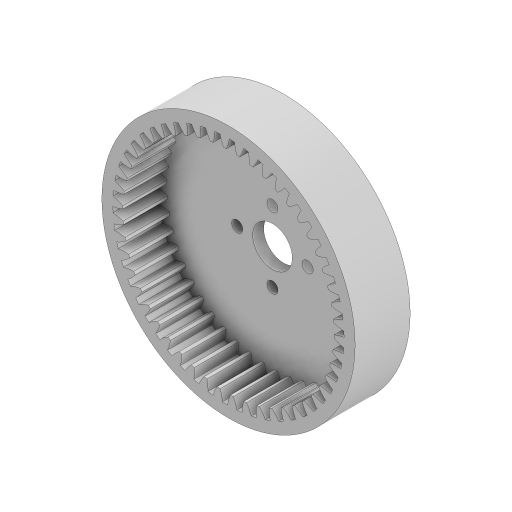
# Autodesk Inventor part: PLANETARIO CORONA
Saved by Autodesk Inventor 2024 (Build 280153000, 153)
## iProperties
Created: 2024-06-18
Part Number: PLANETARIO CORONA
Material: Generic
Document SubType Name: Modeling
Designer: Jhuliams
Density: 1 g/cm^3
Appearance: Default
Author: Jhuliams
Autodesk Inventor part; units mm, degrees
ref_plane "YZ Plane" through (0, 0, 0) normal (1, 0, 0) x (0, 1, 0)
ref_plane "XZ Plane" through (0, 0, 0) normal (0, 1, 0) x (-1, 0, 0)
ref_plane "XY Plane" through (0, 0, 0) normal (0, 0, 1) x (1, 0, 0)
sketch "Sketch1" plane through (0, 0, 0) normal (0, 0, 1) x (1, 0, 0)
  circle A0 centre (0, 0) radius 52.5
  arc A1 (47.9537, -2.1069) -> (47.994, -0.7575) centre (0, 0) ccw
  line L0 (0, 0) -> (74.2646, 0) construction
  line L1 (0, 0) -> (65.7808, 0) construction
  arc A2 (36.3859, -31.306) -> (40.9396, -32.8664) centre (44.1511, -16.0697) ccw
  arc A3 (47.9537, -2.1069) -> (52.3718, -3.6673) centre (55.8044, 13.0856) ccw
  arc A4 (52.4973, 0.5366) -> (47.994, -0.7575) centre (54.9244, -16.3913) ccw
  arc A5 (47.8397, 3.9199) -> (47.7105, 5.2637) centre (0, 0) ccw
  arc A6 (47.8397, 3.9199) -> (52.4184, 2.9255) centre (53.7243, 19.9766) ccw
  arc A7 (52.016, 7.112) -> (47.7105, 5.2637) centre (56.5456, -9.3782) ccw
  arc A8 (46.9711, 9.8849) -> (46.6746, 11.2019) centre (0, 0) ccw
  arc A9 (46.9711, 9.8849) -> (51.6384, 9.4722) centre (50.7969, 26.5525) ccw
  arc A10 (50.7145, 13.5753) -> (46.6746, 11.2019) centre (57.2752, -2.2172) ccw
  arc A11 (45.3619, 15.694) -> (44.9026, 16.9634) centre (0, 0) ccw
  arc A12 (45.3619, 15.694) -> (50.0441, 15.8695) centre (47.0684, 32.7097) ccw
  arc A13 (48.6132, 19.8244) -> (44.9026, 16.9634) centre (57.1014, 4.9787) ccw
  arc A14 (43.0372, 21.2556) -> (42.4224, 22.4575) centre (0, 0) ccw
  arc A15 (43.0372, 21.2556) -> (47.6605, 22.0166) centre (42.5977, 38.351) ccw
  arc A16 (45.7452, 25.761) -> (42.4224, 22.4575) centre (56.0272, 12.0962) ccw
  arc A17 (40.0338, 26.482) -> (39.2732, 27.5973) centre (0, 0) ccw
  arc A18 (40.0338, 26.482) -> (44.5252, 27.8164) centre (37.4551, 43.3875) ccw
  arc A19 (42.1558, 31.2912) -> (39.2732, 27.5973) centre (54.0693, 19.0229) ccw
  arc A20 (36.399, 31.2907) -> (35.5047, 32.3019) centre (0, 0) ccw
  arc A21 (36.399, 31.2907) -> (40.6878, 33.1776) centre (31.7219, 47.7397) ccw
  arc A22 (37.9015, 36.328) -> (35.5047, 32.3019) centre (51.2588, 25.6496) ccw
  arc A23 (32.1902, 35.606) -> (31.1762, 36.4972) centre (0, 0) ccw
  arc A24 (32.1902, 35.606) -> (36.2087, 38.0155) centre (25.4884, 51.3391) ccw
  arc A25 (33.0496, 40.7919) -> (31.1762, 36.4972) centre (47.6398, 31.8717) ccw
  arc A26 (27.4738, 39.3598) -> (26.3561, 40.1168) centre (0, 0) ccw
  arc A27 (27.4738, 39.3598) -> (31.1586, 42.2539) centre (18.8529, 54.1288) ccw
  arc A28 (27.6764, 44.6124) -> (26.3561, 40.1168) centre (43.2696, 37.5913) ccw
  arc A29 (22.3241, 42.4928) -> (21.1203, 43.1037) centre (0, 0) ccw
  arc A30 (22.3241, 42.4928) -> (25.6171, 45.8259) centre (11.9201, 56.0649) ccw
  arc A31 (21.8667, 47.7294) -> (21.1203, 43.1037) centre (38.217, 42.718) ccw
  arc A32 (16.8223, 44.9557) -> (15.5514, 45.4109) centre (0, 0) ccw
  arc A33 (16.8223, 44.9557) -> (19.6716, 48.6752) centre (4.7993, 57.1168) ccw
  arc A34 (15.7122, 50.0937) -> (15.5514, 45.4109) centre (32.5616, 47.171) ccw
  arc A35 (11.0552, 46.7096) -> (9.7373, 47.002) centre (0, 0) ccw
  arc A36 (11.0552, 46.7096) -> (13.4159, 50.7569) centre (-2.3971, 57.2679) ccw
  arc A37 (9.3099, 51.6679) -> (9.7373, 47.002) centre (26.3928, 50.8801) ccw
  arc A38 (5.1138, 47.7268) -> (3.7696, 47.8518) centre (0, 0) ccw
  arc A39 (5.1138, 47.7268) -> (6.9486, 52.0381) centre (-9.5558, 56.5159) ccw
  arc A40 (2.7608, 52.4274) -> (3.7696, 47.8518) centre (19.8077, 53.7868) ccw
  arc A41 (-0.9083, 47.9914) -> (-2.2575, 47.9469) centre (0, 0) ccw
  arc A42 (-0.9083, 47.9914) -> (0.3717, 52.4987) centre (-16.5638, 54.8726) ccw
  arc A43 (-3.8319, 52.36) -> (-2.2575, 47.9469) centre (12.9102, 55.8452) ccw
  arc A44 (-6.9161, 47.4991) -> (-8.2491, 47.2859) centre (0, 0) ccw
  arc A45 (-6.9161, 47.4991) -> (-6.2111, 52.1313) centre (-23.3105, 52.3639) ccw
  arc A46 (-10.3641, 51.4668) -> (-8.2491, 47.2859) centre (5.8092, 57.0229) ccw
  arc A47 (-12.8148, 46.2578) -> (-14.1105, 45.8791) centre (0, 0) ccw
  arc A48 (-12.8148, 46.2578) -> (-12.6959, 50.9418) centre (-29.6897, 49.0294) ccw
  arc A49 (-16.7329, 49.762) -> (-14.1105, 45.8791) centre (-1.3835, 57.3014) ccw
  arc A50 (-18.5113, 44.2869) -> (-19.7494, 43.7488) centre (0, 0) ccw
  arc A51 (-18.5113, 44.2869) -> (-18.9805, 48.9489) centre (-35.6006, 44.9217) ccw
  arc A52 (-22.8378, 47.2725) -> (-19.7494, 43.7488) centre (-8.5543, 56.6761) ccw
  arc A53 (-23.916, 41.6176) -> (-25.0769, 40.9286) centre (0, 0) ccw
  arc A54 (-23.916, 41.6176) -> (-24.9658, 46.184) centre (-40.95, 40.1055) ccw
  arc A55 (-28.5825, 44.0374) -> (-25.0769, 40.9286) centre (-15.5903, 55.1571) ccw
  arc A56 (-28.9435, 38.292) -> (-30.0088, 37.4629) centre (0, 0) ccw
  arc A57 (-28.9435, 38.292) -> (-30.5573, 42.6908) centre (-45.6537, 34.6569) ccw
  arc A58 (-33.8765, 40.1078) -> (-30.0088, 37.4629) centre (-22.3804, 52.7682) ccw
  arc A59 (-33.5145, 34.3624) -> (-34.4676, 33.4064) centre (0, 0) ccw
  arc A60 (-33.5145, 34.3624) -> (-35.6669, 38.5243) centre (-49.6373, 28.6617) ccw
  arc A61 (-38.6362, 35.5457) -> (-34.4676, 33.4064) centre (-28.8175, 49.5471) ccw
  arc A62 (-37.557, 29.891) -> (-38.3827, 28.823) centre (0, 0) ccw
  arc A63 (-37.557, 29.891) -> (-40.214, 33.7503) centre (-52.8382, 22.2145) ccw
  arc A64 (-42.7866, 30.423) -> (-38.3827, 28.823) centre (-34.8002, 45.5446) ccw
  arc A65 (-41.0072, 24.9482) -> (-41.6925, 23.7851) centre (0, 0) ccw
  arc A66 (-41.0072, 24.9482) -> (-44.127, 28.444) centre (-55.2058, 15.4169) ccw
  arc A67 (-46.2622, 24.8205) -> (-41.6925, 23.7851) centre (-40.234, 40.8238) ccw
  arc A68 (-43.8107, 19.6119) -> (-44.3448, 18.3721) centre (0, 0) ccw
  arc A69 (-43.8107, 19.6119) -> (-47.344, 22.6891) centre (-56.7027, 8.3763) ccw
  arc A70 (-49.0082, 18.8266) -> (-44.3448, 18.3721) centre (-45.0333, 35.4593) ccw
  arc A71 (-45.9232, 13.9663) -> (-46.2978, 12.6694) centre (0, 0) ccw
  arc A72 (-45.9232, 13.9663) -> (-49.8144, 16.5764) centre (-57.3054, 1.2035) ccw
  arc A73 (-50.9814, 12.5358) -> (-46.2978, 12.6694) centre (-49.1224, 29.5355) ccw
  arc A74 (-47.3115, 8.1005) -> (-47.5206, 6.7668) centre (0, 0) ccw
  arc A75 (-47.3115, 8.1005) -> (-51.4991, 10.2023) centre (-57.0044, -5.9883) ccw
  arc A76 (-52.1506, 6.0473) -> (-47.5206, 6.7668) centre (-52.4369, 23.1459) ccw
  arc A77 (-47.9537, 2.1069) -> (-47.994, 0.7575) centre (0, 0) ccw
  arc A78 (-47.9537, 2.1069) -> (-52.3718, 3.6673) centre (-55.8044, -13.0856) ccw
  arc A79 (-52.4973, -0.5366) -> (-47.994, 0.7575) centre (-54.9244, 16.3913) ccw
  arc A80 (-47.8397, -3.9199) -> (-47.7105, -5.2637) centre (0, 0) ccw
  arc A81 (-47.8397, -3.9199) -> (-52.4184, -2.9255) centre (-53.7243, -19.9766) ccw
  arc A82 (-52.016, -7.112) -> (-47.7105, -5.2637) centre (-56.5456, 9.3782) ccw
  arc A83 (-46.9711, -9.8849) -> (-46.6746, -11.2019) centre (0, 0) ccw
  arc A84 (-46.9711, -9.8849) -> (-51.6384, -9.4722) centre (-50.7969, -26.5525) ccw
  arc A85 (-50.7145, -13.5753) -> (-46.6746, -11.2019) centre (-57.2752, 2.2172) ccw
  arc A86 (-45.3619, -15.694) -> (-44.9026, -16.9634) centre (0, 0) ccw
  arc A87 (-45.3619, -15.694) -> (-50.0441, -15.8695) centre (-47.0684, -32.7097) ccw
  arc A88 (-48.6132, -19.8244) -> (-44.9026, -16.9634) centre (-57.1014, -4.9787) ccw
  arc A89 (-43.0372, -21.2556) -> (-42.4224, -22.4575) centre (0, 0) ccw
  arc A90 (-43.0372, -21.2556) -> (-47.6605, -22.0166) centre (-42.5977, -38.351) ccw
  arc A91 (-45.7452, -25.761) -> (-42.4224, -22.4575) centre (-56.0272, -12.0962) ccw
  arc A92 (-40.0338, -26.482) -> (-39.2732, -27.5973) centre (0, 0) ccw
  arc A93 (-40.0338, -26.482) -> (-44.5252, -27.8164) centre (-37.4551, -43.3875) ccw
  arc A94 (-42.1558, -31.2912) -> (-39.2732, -27.5973) centre (-54.0693, -19.0229) ccw
  arc A95 (-36.399, -31.2907) -> (-35.5047, -32.3019) centre (0, 0) ccw
  arc A96 (-36.399, -31.2907) -> (-40.6878, -33.1776) centre (-31.7219, -47.7397) ccw
  arc A97 (-37.9015, -36.328) -> (-35.5047, -32.3019) centre (-51.2588, -25.6496) ccw
  arc A98 (-32.1902, -35.606) -> (-31.1762, -36.4972) centre (0, 0) ccw
  arc A99 (-32.1902, -35.606) -> (-36.2087, -38.0155) centre (-25.4884, -51.3391) ccw
  arc A100 (-33.0496, -40.7919) -> (-31.1762, -36.4972) centre (-47.6398, -31.8717) ccw
  arc A101 (-27.4738, -39.3598) -> (-26.3561, -40.1168) centre (0, 0) ccw
  arc A102 (-27.4738, -39.3598) -> (-31.1586, -42.2539) centre (-18.8529, -54.1288) ccw
  arc A103 (-27.6764, -44.6124) -> (-26.3561, -40.1168) centre (-43.2696, -37.5913) ccw
  arc A104 (-22.3241, -42.4928) -> (-21.1203, -43.1037) centre (0, 0) ccw
  arc A105 (-22.3241, -42.4928) -> (-25.6171, -45.8259) centre (-11.9201, -56.0649) ccw
  arc A106 (-21.8667, -47.7294) -> (-21.1203, -43.1037) centre (-38.217, -42.718) ccw
  arc A107 (-16.8223, -44.9557) -> (-15.5514, -45.4109) centre (0, 0) ccw
  arc A108 (-16.8223, -44.9557) -> (-19.6716, -48.6752) centre (-4.7993, -57.1168) ccw
  arc A109 (-15.7122, -50.0937) -> (-15.5514, -45.4109) centre (-32.5616, -47.171) ccw
  arc A110 (-11.0552, -46.7096) -> (-9.7373, -47.002) centre (0, 0) ccw
  arc A111 (-11.0552, -46.7096) -> (-13.4159, -50.7569) centre (2.3971, -57.2679) ccw
  arc A112 (-9.3099, -51.6679) -> (-9.7373, -47.002) centre (-26.3928, -50.8801) ccw
  arc A113 (-5.1138, -47.7268) -> (-3.7696, -47.8518) centre (0, 0) ccw
  arc A114 (-5.1138, -47.7268) -> (-6.9486, -52.0381) centre (9.5558, -56.5159) ccw
  arc A115 (-2.7608, -52.4274) -> (-3.7696, -47.8518) centre (-19.8077, -53.7868) ccw
  arc A116 (0.9083, -47.9914) -> (2.2575, -47.9469) centre (0, 0) ccw
  arc A117 (0.9083, -47.9914) -> (-0.3717, -52.4987) centre (16.5638, -54.8726) ccw
  arc A118 (3.8319, -52.36) -> (2.2575, -47.9469) centre (-12.9102, -55.8452) ccw
  arc A119 (6.9161, -47.4991) -> (8.2491, -47.2859) centre (0, 0) ccw
  arc A120 (6.9161, -47.4991) -> (6.2111, -52.1313) centre (23.3105, -52.3639) ccw
  arc A121 (10.3641, -51.4668) -> (8.2491, -47.2859) centre (-5.8092, -57.0229) ccw
  arc A122 (12.8148, -46.2578) -> (14.1105, -45.8791) centre (0, 0) ccw
  arc A123 (12.8148, -46.2578) -> (12.6959, -50.9418) centre (29.6897, -49.0294) ccw
  arc A124 (16.7329, -49.762) -> (14.1105, -45.8791) centre (1.3835, -57.3014) ccw
  arc A125 (18.5113, -44.2869) -> (19.7494, -43.7488) centre (0, 0) ccw
  arc A126 (18.5113, -44.2869) -> (18.9805, -48.9489) centre (35.6006, -44.9217) ccw
  arc A127 (22.8378, -47.2725) -> (19.7494, -43.7488) centre (8.5543, -56.6761) ccw
  arc A128 (23.916, -41.6176) -> (25.0769, -40.9286) centre (0, 0) ccw
  arc A129 (23.916, -41.6176) -> (24.9658, -46.184) centre (40.95, -40.1055) ccw
  arc A130 (28.5825, -44.0374) -> (25.0769, -40.9286) centre (15.5903, -55.1571) ccw
  arc A131 (28.9435, -38.292) -> (30.0088, -37.4629) centre (0, 0) ccw
  arc A132 (28.9435, -38.292) -> (30.5573, -42.6908) centre (45.6537, -34.6569) ccw
  arc A133 (33.8765, -40.1078) -> (30.0088, -37.4629) centre (22.3804, -52.7682) ccw
  arc A134 (33.5145, -34.3624) -> (34.4676, -33.4064) centre (0, 0) ccw
  arc A135 (33.5145, -34.3624) -> (35.6669, -38.5243) centre (49.6373, -28.6617) ccw
  arc A136 (38.6362, -35.5457) -> (34.4676, -33.4064) centre (28.8175, -49.5471) ccw
  arc A137 (37.557, -29.891) -> (38.3827, -28.823) centre (0, 0) ccw
  arc A138 (37.557, -29.891) -> (40.214, -33.7503) centre (52.8382, -22.2145) ccw
  arc A139 (42.7866, -30.423) -> (38.3827, -28.823) centre (34.8002, -45.5446) ccw
  arc A140 (41.0072, -24.9482) -> (41.6925, -23.7851) centre (0, 0) ccw
  arc A141 (41.0072, -24.9482) -> (44.127, -28.444) centre (55.2058, -15.4169) ccw
  arc A142 (46.2622, -24.8205) -> (41.6925, -23.7851) centre (40.234, -40.8238) ccw
  arc A143 (43.8107, -19.6119) -> (44.3448, -18.3721) centre (0, 0) ccw
  arc A144 (43.8107, -19.6119) -> (47.344, -22.6891) centre (56.7027, -8.3763) ccw
  arc A145 (49.0082, -18.8266) -> (44.3448, -18.3721) centre (45.0333, -35.4593) ccw
  arc A146 (45.9232, -13.9663) -> (46.2978, -12.6694) centre (0, 0) ccw
  arc A147 (45.9232, -13.9663) -> (49.8144, -16.5764) centre (57.3054, -1.2035) ccw
  arc A148 (50.9814, -12.5358) -> (46.2978, -12.6694) centre (49.1224, -29.5355) ccw
  arc A149 (47.3115, -8.1005) -> (47.5206, -6.7668) centre (0, 0) ccw
  arc A150 (47.3115, -8.1005) -> (51.4991, -10.2023) centre (57.0044, 5.9883) ccw
  arc A151 (52.1506, -6.0473) -> (47.5206, -6.7668) centre (52.4369, -23.1459) ccw
  circle A152 centre (0, 0) radius 57.5
  point P0 (52.1506, -6.0473)
  point P1 (51.4991, -10.2023)
  point P2 (47.344, -22.6891)
  point P3 (44.127, -28.444)
  point P4 (38.6362, -35.5457)
  point P5 (30.5573, -42.6908)
  point P6 (28.5825, -44.0374)
  point P7 (24.9658, -46.184)
  point P8 (22.8378, -47.2725)
  point P9 (18.9805, -48.9489)
  point P10 (16.7329, -49.762)
  point P11 (12.6959, -50.9418)
  point P12 (10.3641, -51.4668)
  point P13 (6.2111, -52.1313)
  point P14 (3.8319, -52.36)
  point P15 (-0.3717, -52.4987)
  point P16 (-2.7608, -52.4274)
  point P17 (-6.9486, -52.0381)
  point P18 (-9.3099, -51.6679)
  point P19 (-13.4159, -50.7569)
  point P20 (-25.6171, -45.8259)
  point P21 (-31.1586, -42.2539)
  point P22 (-36.2087, -38.0155)
  point P23 (-40.6878, -33.1776)
  point P24 (-42.1558, -31.2912)
  point P25 (-44.5252, -27.8164)
  point P26 (-45.7452, -25.761)
  point P27 (-47.6605, -22.0166)
  point P28 (-48.6132, -19.8244)
  point P29 (-50.0441, -15.8695)
  point P30 (-50.7145, -13.5753)
  point P31 (-51.6384, -9.4722)
  point P32 (-52.4184, -2.9255)
  point P33 (-52.4973, -0.5366)
  point P34 (-52.3718, 3.6673)
  point P35 (-52.1506, 6.0473)
  point P36 (-51.4991, 10.2023)
  point P37 (-49.8144, 16.5764)
  point P38 (-44.127, 28.444)
  point P39 (-40.214, 33.7503)
  point P40 (-35.6669, 38.5243)
  point P41 (-30.5573, 42.6908)
  point P42 (-18.9805, 48.9489)
  point P43 (-12.6959, 50.9418)
  point P44 (-6.2111, 52.1313)
  point P45 (-3.8319, 52.36)
  point P46 (0.3717, 52.4987)
  point P47 (2.7608, 52.4274)
  point P48 (6.9486, 52.0381)
  point P49 (13.4159, 50.7569)
  point P50 (19.6716, 48.6752)
  point P51 (21.8667, 47.7294)
  point P52 (25.6171, 45.8259)
  point P53 (27.6764, 44.6124)
  point P54 (31.1586, 42.2539)
  point P55 (33.0496, 40.7919)
  point P56 (36.2087, 38.0155)
  point P57 (40.6878, 33.1776)
  point P58 (42.1558, 31.2912)
  point P59 (44.5252, 27.8164)
  point P60 (45.7452, 25.761)
  point P61 (47.6605, 22.0166)
  point P62 (48.6132, 19.8244)
  point P63 (50.0441, 15.8695)
  point P64 (50.7145, 13.5753)
  point P65 (51.6384, 9.4722)
  point P66 (52.4184, 2.9255)
  dimension "d1" = 105
  dimension "d2" = 96
  dimension "d7" = 360
  dimension "d9" = 115
  constraints: 302 point on circle, 152 centre point, 4 end point, 2 coincident, 2 horizontal, 505 other
  measures "d2" diameter of A1
  measures "d9" diameter of A152
extrude "Extrusion1" add sketch "Sketch1" along normal blind 25 contours A0 A3 A1 A4 | A6 A5 A7 A0 | A0 A150 A149 A151 | A9 A8 A10 A0 | A0 A147 A146 A148 | A12 A11 A13 A0 | A0 A144 A143 A145 | A15 A14 A16 A0 | A0 A141 A140 A142 | A18 A17 A19 A0 | A0 A2 A138 A137 A139 | A0 A138 A2 | A21 A20 A22 A0 | A0 A135 A134 A136 | A24 A23 A25 A0 | A0 A132 A131 A133 | A27 A26 A28 A0 | A0 A129 A128 A130 | A30 A29 A31 A0 | A0 A126 A125 A127 | A33 A32 A34 A0 | A0 A123 A122 A124 | A36 A35 A37 A0 | A0 A120 A119 A121 | A39 A38 A40 A0 | A0 A117 A116 A118 | A42 A41 A43 A0 | A0 A114 A113 A115 | A45 A44 A46 A0 | A0 A111 A110 A112 | A48 A47 A49 A0 | A0 A108 A107 A109 | A51 A50 A52 A0 | A0 A105 A104 A106 | A54 A53 A55 A0 | A0 A102 A101 A103 | A57 A56 A58 A0 | A0 A99 A98 A100 | A60 A59 A61 A0 | A0 A96 A95 A97 | A63 A62 A64 A0 | A0 A93 A92 A94 | A66 A65 A67 A0 | A0 A90 A89 A91 | A69 A68 A70 A0 | A0 A87 A86 A88 | A72 A71 A73 A0 | A0 A84 A83 A85 | A75 A74 A76 A0 | A0 A81 A80 A82 | A78 A77 A79 A0 | A152
sketch "Sketch2" plane through (0, 0, 0) normal (0, 0, -1) x (-1, 0, 0)
  circle A0 centre (0, 0) radius 57.5
  dimension "d12" = 115
  constraints: 1 centre point, 1 coincident
  measures "d12" diameter of A0
extrude "Extrusion2" add sketch "Sketch2" against normal blind 5
sketch "Sketch3" plane through (0, 0, 0) normal (0, 0, -1) x (-1, 0, 0)
  circle A0 centre (0, 0) radius 9
  dimension "d15" = 18
  constraints: 1 centre point, 1 coincident
  measures "d15" diameter of A0
extrude "Extrusion3" cut sketch "Sketch3" against normal blind 5
sketch "Sketch4" plane through (0, 0, 0) normal (0, 0, -1) x (-1, 0, 0)
  circle A0 centre (0, 0) radius 16
  circle A1 centre (16, 0) radius 2.5
  circle A2 centre (0, 16) radius 2.5
  circle A3 centre (-16, 0) radius 2.5
  circle A4 centre (0, -16) radius 2.5
  dimension "d18" = 32
  dimension "d19" = 5
  dimension "d22" = 360
  constraints: 4 centre point, 1 coincident, 1 horizontal alignment, 11 other
  measures "d19" diameter of A1
extrude "Extrusion4" cut sketch "Sketch4" against normal blind 5 contours A0 A1 | A0 A1 | A2 A0 | A0 A2 | A4 A0 | A0 A4 | A3 A0 | A0 A3
body "Solid1"
